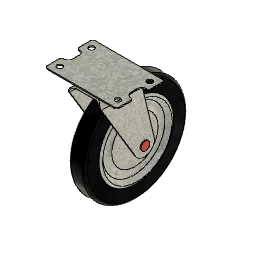
model (Autodesk Fusion 360 archive; units mm, degrees)
design "caster"
Autodesk Fusion 360 part; units mm, degrees
note: some values were not read from the file. Chosen so that the rebuilt part matches the saved one: which bodies a step acts on. Set by a fixed rule: which sketch regions a step uses.
sketch "Sketch1" plane through (0, 0, -18) normal (0, 0, -1) x (1, 0, 0)
  line L0 (0, 0) -> (0, -896)
  line L1 (0, -896) -> (608, -896)
  line L2 (608, -896) -> (608, 0)
  line L3 (608, 0) -> (0, 0)
  line L4 (601, -891) -> (539, -891)
  line L5 (537, -889) -> (537, -878.3333)
  line L6 (539, -876.3333) -> (539.3333, -876.3333)
  line L7 (543.3333, -872.3333) -> (543.3333, -866.1272)
  line L8 (539.3333, -862.1272) -> (538.982, -862.1272)
  line L9 (536.982, -860.1272) -> (536.982, -849.0014)
  line L10 (538.982, -847.0014) -> (600.9814, -847.0014)
  line L11 (602.9814, -849.0014) -> (602.9814, -860.127)
  line L12 (600.9814, -862.127) -> (600.6667, -862.127)
  line L13 (596.6667, -866.127) -> (596.6667, -872.3333)
  line L14 (600.6667, -876.3333) -> (601, -876.3333)
  line L15 (603, -878.3333) -> (603, -889)
  line L16 (603, -883.6667) -> (596.6667, -883.6667) construction
  line L17 (596.6667, -883.6667) -> (596.6667, -876.3333) construction
  arc A0 (596.6667, -872.3333) -> (600.6667, -876.3333) centre (600.6667, -872.3333) ccw
  arc A1 (600.6667, -862.127) -> (596.6667, -866.127) centre (600.6667, -866.127) ccw
  arc A2 (539.3333, -876.3333) -> (543.3333, -872.3333) centre (539.3333, -872.3333) ccw
  arc A3 (543.3333, -866.1272) -> (539.3333, -862.1272) centre (539.3333, -866.1272) ccw
  arc A4 (601, -891) -> (603, -889) centre (601, -889) ccw
  arc A5 (603, -878.3333) -> (601, -876.3333) centre (601, -878.3333) ccw
  arc A6 (537, -889) -> (539, -891) centre (539, -889) ccw
  arc A7 (539, -876.3333) -> (537, -878.3333) centre (539, -878.3333) ccw
  arc A8 (536.982, -860.1272) -> (538.982, -862.1272) centre (538.982, -860.1272) ccw
  arc A9 (538.982, -847.0014) -> (536.982, -849.0014) centre (538.982, -849.0014) ccw
  arc A10 (602.9814, -849.0014) -> (600.9814, -847.0014) centre (600.9814, -849.0014) ccw
  arc A11 (600.9814, -862.127) -> (602.9814, -860.127) centre (600.9814, -860.127) ccw
  point P0 (603, -891)
  dimension "d632" = 5
  dimension "d633" = 5
  dimension "d634" = 4
  dimension "d635" = 2
  constraint perpendicular L4 L5
  constraint perpendicular L5 L6
  constraint perpendicular L6 L7
  constraint perpendicular L7 L8
  constraint perpendicular L8 L9
  constraint perpendicular L9 L10
  constraint perpendicular L10 L11
  constraint perpendicular L11 L12
  constraint perpendicular L12 L13
  constraint perpendicular L13 L14
  constraint perpendicular L4 L15
  constraint perpendicular L15 L16
  constraint perpendicular L16 L17
  constraint coincident L17.end L14
  constraint coincident L17.end L13
  constraint tangent L14 A0
  constraint tangent L13 A0
  constraint tangent L12 A1
  constraint tangent L13 A1
  constraint equal A0 A1
  constraint tangent L6 A2
  constraint tangent L7 A2
  constraint equal A0 A2
  constraint tangent L7 A3
  constraint tangent L8 A3
  constraint equal A0 A3
  constraint coincident L15 L16.start
  constraint coincident P0 L4
  constraint coincident P0 L15
  constraint tangent L4 A4
  constraint tangent L15 A4
  constraint tangent L14 A5
  constraint tangent L15 A5
  constraint equal A4 A5
  constraint tangent L4 A6
  constraint tangent L5 A6
  constraint equal A4 A6
  constraint tangent L5 A7
  constraint tangent L6 A7
  constraint equal A4 A7
  constraint tangent L8 A8
  constraint tangent L9 A8
  constraint equal A4 A8
  constraint tangent L9 A9
  constraint tangent L10 A9
  constraint equal A4 A9
  constraint tangent L10 A10
  constraint tangent L11 A10
  constraint equal A4 A10
  constraint tangent L11 A11
  constraint tangent L12 A11
  constraint equal A4 A11
  measures "d632" horizontal distance of L1.end P0
  measures "d633" vertical distance of L1.end P0
  measures "d634" radius of A0
  measures "d635" radius of A4
extrude "Extrude1" add sketch "Sketch1" along normal blind 1 contours L4 L5 L6 L7 L8 L9 L10 L11 L12 L13 L14 L15 A0 A1 A2 A3 A4 A5 A6 A7 A8 A9 A10 A11 makes body 1
sketch "Sketch2" plane through (0, 0, -19) normal (0, 0, -1) x (1, 0, 0)
  line L0 (600.6667, -862.127) -> (600.9814, -862.127)
  arc A0 (600.9814, -862.127) -> (602.9814, -860.127) centre (600.9814, -860.127) ccw
  line L1 (602.9814, -860.127) -> (602.9814, -849.0014)
  arc A1 (602.9814, -849.0014) -> (600.9814, -847.0014) centre (600.9814, -849.0014) ccw
  line L2 (600.9814, -847.0014) -> (538.982, -847.0014)
  arc A2 (538.982, -847.0014) -> (536.982, -849.0014) centre (538.982, -849.0014) ccw
  line L3 (536.982, -849.0014) -> (536.982, -860.1272)
  arc A3 (536.982, -860.1272) -> (538.982, -862.1272) centre (538.982, -860.1272) ccw
  line L4 (538.982, -862.1272) -> (539.3333, -862.1272)
  arc A4 (543.3333, -866.1272) -> (539.3333, -862.1272) centre (539.3333, -866.1272) ccw
  line L5 (543.3333, -866.1272) -> (543.3333, -872.3333)
  arc A5 (539.3333, -876.3333) -> (543.3333, -872.3333) centre (539.3333, -872.3333) ccw
  line L6 (539.3333, -876.3333) -> (539, -876.3333)
  arc A6 (539, -876.3333) -> (537, -878.3333) centre (539, -878.3333) ccw
  line L7 (537, -878.3333) -> (537, -889)
  arc A7 (537, -889) -> (539, -891) centre (539, -889) ccw
  line L8 (539, -891) -> (601, -891)
  arc A8 (601, -891) -> (603, -889) centre (601, -889) ccw
  line L9 (603, -889) -> (603, -878.3333)
  arc A9 (603, -878.3333) -> (601, -876.3333) centre (601, -878.3333) ccw
  line L10 (601, -876.3333) -> (600.6667, -876.3333)
  arc A10 (596.6667, -872.3333) -> (600.6667, -876.3333) centre (600.6667, -872.3333) ccw
  line L11 (596.6667, -872.3333) -> (596.6667, -866.127)
  arc A11 (600.6667, -862.127) -> (596.6667, -866.127) centre (600.6667, -866.127) ccw
  circle A12 centre (570, -869.0007) radius 15
  line L12 (570, -869.0007) -> (569.9817, -847.0014) construction
  line L13 (570, -869.0007) -> (543.3333, -869.2303) construction
  line L14 (596.6667, -869.2302) -> (570, -869.0007) construction
  line L15 (570, -869.0007) -> (570, -891) construction
  circle A13 centre (570, -869.0007) radius 12
  circle A14 centre (570, -869.0007) radius 9
  dimension "d638" = 30
  dimension "d639" = 24
  dimension "d640" = 18
  constraint coincident A12.centre L12.start
  constraint midpoint L2 L12.end
  constraint midpoint L5 L13.end
  constraint midpoint L11 L14.start
  constraint midpoint L8 L15.end
  constraint equal L13 L14
  constraint equal L12 L15
  constraint concentric A12 A13
  constraint concentric A12 A14
  measures "d638" diameter of A12
  measures "d639" diameter of A13
  measures "d640" diameter of A14
extrude "Extrude2" add sketch "Sketch2" along normal blind 1 separate body contours A13 makes body 2
extrude "Extrude3" add sketch "Sketch2" along normal blind 2 contours A12 | A14 bodies 1 2
extrude "Extrude4" add 1 faces at (571.5, 869.7825, -21) along direction (0, 0, -1) blind 1.5 draft -45 on bodies 1 bodies 1
extrude "Extrude5" add 1 faces at (566.3407, 870.7011, -22.5) along direction (0, 0, -1) blind 2 draft 45 separate body on bodies 1 makes body 3
ref_plane "WorkPlane1" through (570, 869.0007, -23.5) normal (1, 0, 0) x (0, 0, -1)
sketch "Sketch3" plane through (570, 869.0007, -23.5) normal (1, 0, 0) x (0, 1, 0)
  line L0 (18.7238, -4.0657) -> (30.3196, -52.3365)
  arc A0 (13.3916, -59.3001) -> (30.3196, -52.3365) centre (21.3133, -54.5) ccw
  line L1 (13.3916, -59.3001) -> (-18.2554, -7.0729)
  circle A1 centre (21.3133, -54.5) radius 40
  line L2 (9.5, -1) -> (-9.5, -1) construction
  line L3 (-4.9816, -1) -> (5.1631, -1) construction
  arc A2 (-14.8345, -1) -> (-18.2554, -7.0729) centre (-14.8345, -5) ccw
  arc A3 (18.7238, -4.0657) -> (14.8345, -1) centre (14.8345, -5) ccw
  line L4 (-14.8345, -1) -> (-9.5, -1)
  line L5 (9.5, -1) -> (14.8345, -1)
  circle A4 centre (21.3133, -54.5) radius 4
  line L6 (-9.5, -1) -> (9.5, -1)
  point P0 (26.9993, 5.5)
  dimension "d650" = 80
  dimension "d652" = 60
  dimension "d653" = 4
  dimension "d654" = 4
  dimension "d655" = 8
  constraint tangent L0 A0
  constraint tangent A0 L1
  constraint concentric A0 A1
  constraint coincident L2 L3.start
  constraint coincident L2 L3.end
  constraint tangent L1 A2
  constraint tangent L0 A3
  constraint coincident L2.end L4.end
  constraint parallel L2 L4
  constraint coincident L2.start L5.start
  constraint tangent A3 L5
  constraint tangent A2 L4
  constraint equal L4 L5
  constraint collinear L4 L5
  constraint concentric A0 A4
  measures "d650" diameter of A1
  measures "d652" vertical distance of A0.centre P0
  measures "d653" radius of A2
  measures "d654" radius of A3
  measures "d655" diameter of A4
ref_plane "WorkPlane2" through (570, 869.0007, -23.5) normal (0, 1, 0) x (0, 0, -1)
sketch "Sketch4" plane through (570, 869.0007, -23.5) normal (0, 1, 0) x (1, 0, 0)
  line L0 (9, 1) -> (-9, 1)
  line L1 (-15, 7) -> (-15, 78.4318)
  line L2 (-15, 78.4318) -> (15, 78.4318)
  line L3 (15, 78.4318) -> (15, 7)
  line L4 (0, 14.5) -> (0, 94.5) construction
  line L5 (15, 23.473) -> (0, 23.473) construction
  line L6 (0, 23.473) -> (-15, 23.473) construction
  line L7 (-15, -2.5) -> (-15, 1) construction
  arc A0 (9, 1) -> (15, 7) centre (9, 7) ccw
  arc A1 (-15, 7) -> (-9, 1) centre (-9, 7) ccw
  arc A2 (9, 2) -> (14, 7) centre (9, 7) ccw
  line L8 (14, 77.4318) -> (14, 7)
  line L9 (-14, 77.4318) -> (14, 77.4318)
  line L10 (-14, 7) -> (-14, 77.4318)
  arc A3 (-14, 7) -> (-9, 2) centre (-9, 7) ccw
  line L11 (9, 2) -> (-9, 2)
  point P0 (-15, -2.5)
  point P1 (0, 1)
  dimension "d657" = 6
  dimension "d658" = 1
  constraint horizontal L0
  constraint vertical L1
  constraint horizontal L2
  constraint vertical L3
  constraint coincident L3 L5.start
  constraint coincident L4 L5.end
  constraint perpendicular L3 L5
  constraint coincident L1 L6.end
  constraint perpendicular L1 L6
  constraint equal L5 L6
  constraint coincident P0 L7.start
  constraint vertical L7
  constraint coincident L0 P1
  constraint tangent L0 A0
  constraint tangent L3 A0
  constraint coincident L7.end L0
  constraint coincident L7.end L1
  constraint tangent L0 A1
  constraint tangent L1 A1
  constraint equal A0 A1
  measures "d657" radius of A0
extrude "Extrude6" add sketch "Sketch4" along normal mid plane 200 separate body makes body 4
extrude "Extrude7" add sketch "Sketch3" along normal up to surface (15 mm away) and the other way up to surface (15 mm away) separate body contours L0 L1 A1 A2 A3 L4 L5 L6 | L0 A0 L1 A1 picked at (8.1089, -46.0283) makes body 5
combine "Combine1" operation intersect target body 4 tool bodies 5
ref_plane "WorkPlane3" through (598.5, 890.314, -78) normal (0, -1, 0) x (1, 0, 0)
sketch "Sketch5" plane through (598.5, 890.314, -78) normal (0, -1, 0) x (1, 0, 0)
  line L0 (-28.5, 40) -> (-28.5, -40)
  line L1 (-28.5, 34.268) -> (-20.9325, 34.268)
  line L2 (-20.9325, 34.268) -> (-20.9325, 44.8259)
  line L3 (-28.5, -4.8001) -> (-28.5, 47.4271)
  arc A0 (-20.9325, 44.8259) -> (-23.5336, 47.4271) centre (-23.5336, 44.8259) ccw
  line L4 (-20.9325, 34.268) -> (-19.8153, 31.892)
  line L5 (-19.8153, 31.892) -> (-23.138, 28.4976)
  arc A1 (-23.138, 28.4976) -> (-22.1041, 21.2349) centre (-19.8337, 25.2631) ccw
  line L6 (-22.1041, 21.2349) -> (-22.1041, 6.0645)
  line L7 (-22.1041, 6.0645) -> (-17.674, 3.5615)
  line L8 (-17.674, 3.5615) -> (-17.674, 0)
  line L9 (-17.674, 0) -> (-28.5, 0)
  line L10 (-28.5, 47.4271) -> (-33.3217, 47.4271) construction
  line L11 (-28.5, 47.4271) -> (-23.5336, 47.4271)
  point P0 (-28.5, 0)
  constraint coincident L0 L1.start
  constraint perpendicular L0 L1
  constraint perpendicular L1 L2
  constraint tangent L2 A0
  constraint tangent L5 A1
  constraint perpendicular L1 L6
  constraint perpendicular L1 L8
  constraint coincident P0 L9.end
  constraint perpendicular L8 L9
  constraint perpendicular L3 L10
  constraint coincident L3.end L10.start
  constraint tangent A0 L11
  constraint perpendicular L2 L11
revolve "Revolve1" add sketch "Sketch5" angle 360 about axis through (597.5, 890.314, -78) along (1, 0, 0) separate body contours L0 L1 L3 L4 L5 A1 L6 L7 L8 L9 makes body 6
revolve "Revolve2" add sketch "Sketch5" angle 360 about axis through (597.5, 890.314, -78) along (1, 0, 0) separate body contours L0 L1 L2 L3 A0 L11 makes body 7
ref_plane "WorkPlane4" through (570, 890.314, -78) normal (-1, 0, 0) x (0, 0, 1)
mirror "Mirror1" about plane through (570, 890.314, -78) normal (-1, 0, 0) of bodies 7 6 makes body 8 at (570, 893.6809, -67.0848) makes body 9 at (562.4325, 894.2434, -36.9878)
extrude "Extrude8" add sketch "Sketch3" along normal up to surface (16 mm away) and the other way up to surface (16 mm away) separate body contours A4 makes body 10
sketch "Sketch6" plane through (0, 0, -19) normal (0, 0, -1) x (1, 0, 0)
  circle A0 centre (570, -869.0007) radius 15
  line L0 (600.6667, -862.127) -> (600.9814, -862.127)
  arc A1 (600.9814, -862.127) -> (602.9814, -860.127) centre (600.9814, -860.127) ccw
  line L1 (602.9814, -860.127) -> (602.9814, -849.0014)
  arc A2 (602.9814, -849.0014) -> (600.9814, -847.0014) centre (600.9814, -849.0014) ccw
  line L2 (600.9814, -847.0014) -> (538.982, -847.0014)
  arc A3 (538.982, -847.0014) -> (536.982, -849.0014) centre (538.982, -849.0014) ccw
  line L3 (536.982, -849.0014) -> (536.982, -860.1272)
  arc A4 (536.982, -860.1272) -> (538.982, -862.1272) centre (538.982, -860.1272) ccw
  line L4 (538.982, -862.1272) -> (539.3333, -862.1272)
  arc A5 (543.3333, -866.1272) -> (539.3333, -862.1272) centre (539.3333, -866.1272) ccw
  line L5 (543.3333, -866.1272) -> (543.3333, -872.3333)
  arc A6 (539.3333, -876.3333) -> (543.3333, -872.3333) centre (539.3333, -872.3333) ccw
  line L6 (539.3333, -876.3333) -> (539, -876.3333)
  arc A7 (539, -876.3333) -> (537, -878.3333) centre (539, -878.3333) ccw
  line L7 (537, -878.3333) -> (537, -889)
  arc A8 (537, -889) -> (539, -891) centre (539, -889) ccw
  line L8 (539, -891) -> (601, -891)
  arc A9 (601, -891) -> (603, -889) centre (601, -889) ccw
  line L9 (603, -889) -> (603, -878.3333)
  arc A10 (603, -878.3333) -> (601, -876.3333) centre (601, -878.3333) ccw
  line L10 (601, -876.3333) -> (600.6667, -876.3333)
  arc A11 (596.6667, -872.3333) -> (600.6667, -876.3333) centre (600.6667, -872.3333) ccw
  line L11 (596.6667, -872.3333) -> (596.6667, -866.127)
  arc A12 (600.6667, -862.127) -> (596.6667, -866.127) centre (600.6667, -866.127) ccw
  circle A13 centre (596.6667, -883.6667) radius 2.5
  circle A14 centre (543.3333, -883.6667) radius 2.5
  circle A15 centre (543.3333, -854.3347) radius 2.5
  circle A16 centre (596.6667, -854.3347) radius 2.5
  line L12 (596.6667, -883.6667) -> (596.6667, -854.3347) construction
  line L13 (596.6667, -854.3347) -> (543.3333, -854.3347) construction
  line L14 (543.3333, -854.3347) -> (543.3333, -883.6667) construction
  line L15 (543.3333, -883.6667) -> (596.6667, -883.6667) construction
  line L16 (543.3333, -872.3333) -> (543.3333, -866.1272) construction
  line L17 (596.6667, -883.6667) -> (596.6667, -891) construction
  line L18 (596.6667, -854.3347) -> (596.6667, -847.0014) construction
  point P0 (596.6667, -883.6667)
  dimension "d675" = 5
  dimension "d676" = 5
  dimension "d677" = 5
  dimension "d678" = 5
  constraint coincident P0 A13.centre
  constraint coincident A16.centre L12.end
  constraint coincident A15.centre L13.end
  constraint coincident A14.centre L14.end
  constraint perpendicular L12 L15
  constraint perpendicular L14 L15
  constraint perpendicular L13 L14
  constraint collinear L14 L16
  constraint coincident L8 L17.end
  constraint perpendicular L8 L17
  constraint coincident L2 L18.end
  constraint perpendicular L2 L18
  constraint equal L17 L18
  measures "d675" diameter of A13
  measures "d676" diameter of A14
  measures "d677" diameter of A15
  measures "d678" diameter of A16
extrude "Extrude9" cut sketch "Sketch6" against normal blind 1 contours A13 | A14 | A15 | A16 bodies 1
move_body "Move1" bodies 1 8 9 3 4 6 7 10 to x (1, 0, 0) y (0, 1, 0) z (0, 0, 1) at (-538.982, -847.0014, 18)
combine "Combine2" operation add target body 6 tool bodies 8
combine "Combine3" operation add target body 7 tool bodies 9
equation "d650 = casterDiameter"
equation "d652 = casterTotalHeight - ( casterDiameter / 2 )"
equation "d676 = d675"
equation "d677 = d676"
equation "d678 = d675"
equation "casterDiameter = 80 mm"
equation "casterTotalHeight = 100 mm"
named bodies: "plate", "wheel bearing", "wheel support", "mag", "tire", "axle"
